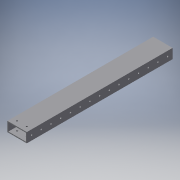
# Autodesk Inventor part: Vertical_intake_frame
Saved by Autodesk Inventor 2018 (Build 220112000, 112)
## iProperties
Created: 2018-09-06
Part Number: Vertical_intake_frame
Material: Generic
Document SubType Name: Modeling
Designer: baoan
Density: 1 g/cm^3
Appearance: Default
Author: baoan
Autodesk Inventor part; units mm, degrees
ref_plane "YZ Plane" through (0, 0, 0) normal (1, 0, 0) x (0, 1, 0)
ref_plane "XZ Plane" through (0, 0, 0) normal (0, 1, 0) x (-1, 0, 0)
ref_plane "XY Plane" through (0, 0, 0) normal (0, 0, 1) x (1, 0, 0)
sketch "Sketch1" plane through (0, 0, 0) normal (0, 0, 1) x (1, 0, 0)
  line L0 (-25.4, -12.7) -> (25.4, -12.7)
  line L1 (25.4, -12.7) -> (25.4, 12.7)
  line L2 (25.4, 12.7) -> (-25.4, 12.7)
  line L3 (-25.4, 12.7) -> (-25.4, -12.7)
  line L4 (-25.4, -12.7) -> (25.4, 12.7) construction
  line L5 (25.4, -12.7) -> (-25.4, 12.7) construction
  line L6 (-22.86, -10.16) -> (22.86, -10.16)
  line L7 (22.86, -10.16) -> (22.86, 10.16)
  line L8 (22.86, 10.16) -> (-22.86, 10.16)
  line L9 (-22.86, 10.16) -> (-22.86, -10.16)
  line L10 (-22.86, -10.16) -> (22.86, 10.16) construction
  line L11 (22.86, -10.16) -> (-22.86, 10.16) construction
  point P0 (0, 0)
  dimension "d0" = 50.8
  dimension "d1" = 25.4
  dimension "d2" = 45.72
  dimension "d3" = 20.32
  constraints: 24 end point, 4 midpoint, 4 parallel, 2 horizontal, 2 perpendicular
  measures "d0" distance of L2.end L1.end
  measures "d1" distance of L1.end L0.end
  measures "d2" distance of L8.end L7.end
  measures "d3" distance of L7.end L6.end
extrude "Extrusion1" add sketch "Sketch1" along normal mid plane 381
sketch "Sketch2" plane through (25.4, -12.7, 190.5) normal (1, 0, 0) x (0, 0, -1)
  line L0 (381, 25.4) -> (0, 25.4) projected
  line L1 (0, 0) -> (0, 25.4) projected
  point P0 (190.5, 12.7)
  point P1 (12.7, 12.7)
  dimension "d6" = 12.7
  dimension "d7" = 12.7
  measures "d6" distance from line of L0 point (12.7, 12.7)
  measures "d7" distance from line of L1 point (12.7, 12.7)
hole "Hole1" at (25.4, 0, 177.8) direction (-1, 0, 0) diameter 4.1402 end through all
pattern_linear "Rectangular Pattern1" count 15 spacing 25.4 along (0, 0, -1) of "Hole1"
sketch "Sketch4" plane through (-25.4, -12.7, 190.5) normal (0, -1, 0) x (1, 0, 0)
  line L0 (0, 0) -> (50.8, 0) projected
  line L1 (50.8, -381) -> (50.8, 0) projected
  point P0 (25.4, -190.5)
  point P1 (38.1, -19.05)
  point P2 (12.7, -19.05)
  dimension "d38" = 25.4
  dimension "d39" = 19.05
  dimension "d40" = 12.7
  constraints: 1 horizontal alignment
  measures "d38" distance of point (38.1, -19.05) point (12.7, -19.05)
  measures "d39" distance from line of L0 point (38.1, -19.05)
  measures "d40" distance from line of L1 point (38.1, -19.05)
hole "Hole4" at (12.7, -12.7, 171.45) at (-12.7, -12.7, 171.45) direction (0, 1, 0) diameter 4.1402 end through all
body "Solid1"
